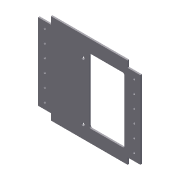
# Autodesk Inventor part: DriveTrain_MotorMount
Saved by Autodesk Inventor 2012 (Build 160160000, 160)
## iProperties
Created: 2012-01-08
Part Number: DriveTrain_MotorMount
Material: Aluminum-6061
Document SubType Name: Modeling
Designer: JesseK
Density: 2.71 g/cm^3
Mass: 300.27 g
Surface Area: 729.239 cm^2
Volume: 110.801 cm^3
Author: JesseK
Autodesk Inventor part; units mm, degrees
ref_plane "YZ Plane" through (0, 0, 0) normal (1, 0, 0) x (0, 1, 0)
ref_plane "XZ Plane" through (0, 0, 0) normal (0, 1, 0) x (-1, 0, 0)
ref_plane "XY Plane" through (0, 0, 0) normal (0, 0, 1) x (1, 0, 0)
sketch "Sketch1" plane through (0, 0, 0) normal (0, 0, 1) x (1, 0, 0)
  line L0 (203.2, 0) -> (203.2, 154.2919)
  line L1 (0, 152.4) -> (0, 0)
  line L2 (177.8, 154.2919) -> (177.8, 166.9919)
  line L3 (177.8, 166.9919) -> (25.4, 166.9919)
  line L4 (25.4, 166.9919) -> (25.4, 152.4)
  line L5 (0, 152.4) -> (25.4, 152.4)
  line L6 (177.8, 154.2919) -> (203.2, 154.2919)
  line L7 (177.8, 0) -> (177.8, -12.7)
  line L8 (177.8, -12.7) -> (25.4, -12.7)
  line L9 (25.4, -12.7) -> (25.4, 0)
  line L10 (0, 0) -> (25.4, 0)
  line L11 (177.8, 0) -> (203.2, 0)
  dimension "d0" = 152.4
  dimension "d1" = 203.2
  dimension "d18" = 25.4
  dimension "d19" = 25.4
  dimension "d20" = 12.7
  dimension "d21" = 25.4
  dimension "d22" = 25.4
  dimension "d23" = 12.7
  constraints: 24 end point, 4 parallel, 1 collinear, 1 perpendicular
  measures "d0" distance of L1.start L1.end
  measures "d1" distance of L1.end L0.start
  measures "d18" distance between parallel lines of L1 L4
  measures "d19" distance between parallel lines of L0 L2
  measures "d20" distance of L2.start L2.end
  measures "d21" distance of L1.end L9.end
  measures "d22" distance of L7.start L0.start
  measures "d23" distance of L7.start L7.end
extrude "Extrusion3" add sketch "Sketch1" along normal blind 3.175
sketch "Sketch2" plane through (0, 0, 3.175) normal (0, 0, 1) x (1, 0, 0)
  line L0 (0, 152.4) -> (25.4, 152.4) projected
  line L1 (0, 0) -> (0, 152.4) projected
  line L2 (25.4, 0) -> (0, 0) projected
  line L3 (203.2, 0) -> (177.8, 0) projected
  line L4 (177.8, 154.2919) -> (203.2, 154.2919) projected
  line L5 (25.4, 152.4) -> (25.4, 166.9919) projected
  line L6 (12.7, 152.4) -> (12.7, 139.7) construction
  line L7 (12.7, 139.7) -> (12.7, 114.3) construction
  line L8 (12.7, 114.3) -> (12.7, 88.9) construction
  line L9 (12.7, 88.9) -> (12.7, 63.5) construction
  line L10 (12.7, 63.5) -> (12.7, 38.1) construction
  line L11 (12.7, 38.1) -> (12.7, 12.7) construction
  line L12 (12.7, 12.7) -> (12.7, 0) construction
  circle A0 centre (12.7, 139.7) radius 2.3813
  circle A1 centre (12.7, 114.3) radius 2.3813
  circle A2 centre (12.7, 88.9) radius 2.3813
  circle A3 centre (12.7, 63.5) radius 2.3813
  circle A4 centre (12.7, 38.1) radius 2.3813
  circle A5 centre (12.7, 12.7) radius 2.3813
  line L13 (190.5, 154.2919) -> (190.5, 141.5919) construction
  line L14 (190.5, 141.5919) -> (190.5, 116.1919) construction
  line L15 (190.5, 116.1919) -> (190.5, 90.7919) construction
  line L16 (190.5, 90.7919) -> (190.5, 65.3919) construction
  line L17 (190.5, 65.3919) -> (190.5, 39.9919) construction
  line L18 (190.5, 39.9919) -> (190.5, 14.5919) construction
  line L19 (190.5, 14.5919) -> (190.5, 0) construction
  circle A6 centre (190.5, 141.5919) radius 2.3813
  circle A7 centre (190.5, 116.1919) radius 2.3813
  circle A8 centre (190.5, 90.7919) radius 2.3813
  circle A9 centre (190.5, 65.3919) radius 2.3813
  circle A10 centre (190.5, 39.9919) radius 2.3813
  circle A11 centre (190.5, 14.5919) radius 2.3813
  dimension "d26" = 12.7
  dimension "d27" = 25.4
  dimension "d28" = 4.7625
  dimension "d29" = 12.7
  dimension "d30" = 25.4
  dimension "d31" = 4.7625
  constraints: 28 end point, 18 collinear, 12 centre point, 12 coincident, 10 equal radius, 4 midpoint, 3 parallel
  measures "d26" distance of L6.start L6.end
  measures "d27" distance of L6.end L7.end
  measures "d28" diameter of A2
  measures "d29" distance of L13.start L13.end
  measures "d30" distance of L13.end L14.end
  measures "d31" diameter of A6
extrude "Extrusion4" cut sketch "Sketch2" against normal up to next
sketch "Sketch3" plane through (0, 0, 3.175) normal (0, 0, 1) x (1, 0, 0)
  line L0 (0, 0) -> (0, 152.4) projected
  line L1 (25.4, 0) -> (0, 0) projected
  circle A0 centre (88.9, 127) radius 3.175
  circle A1 centre (88.9, 12.7) radius 3.175
  dimension "d34" = 88.9
  dimension "d35" = 88.9
  dimension "d36" = 114.3
  dimension "d37" = 12.7
  dimension "d38" = 6.35
  dimension "d39" = 6.35
  constraints: 2 centre point
  measures "d34" distance from line of A0.centre L0
  measures "d35" distance from line of L0 A1.centre
  measures "d36" distance of A0.centre A1.centre
  measures "d37" distance from line of L1 A1.centre
  measures "d38" diameter of A0
  measures "d39" diameter of A1
extrude "Extrusion5" cut sketch "Sketch3" against normal up to next
sketch "Sketch4" plane through (0, 0, 3.175) normal (0, 0, 1) x (1, 0, 0)
  circle A0 centre (88.9, 127) radius 3.175 projected
  line L0 (203.2, 0) -> (177.8, 0) projected
  line L1 (203.2, 154.2919) -> (203.2, 0) projected
  line L2 (177.8, 154.2919) -> (203.2, 154.2919) projected
  line L3 (104.775, 141.5919) -> (168.275, 141.5919)
  line L4 (171.45, 138.4169) -> (171.45, 15.875)
  line L5 (168.275, 12.7) -> (104.775, 12.7)
  line L6 (101.6, 15.875) -> (101.6, 138.4169)
  arc A1 (104.775, 141.5919) -> (101.6, 138.4169) centre (104.775, 138.4169) ccw
  arc A2 (171.45, 138.4169) -> (168.275, 141.5919) centre (168.275, 138.4169) ccw
  arc A3 (168.275, 12.7) -> (171.45, 15.875) centre (168.275, 15.875) ccw
  arc A4 (101.6, 15.875) -> (104.775, 12.7) centre (104.775, 15.875) ccw
  dimension "d42" = 12.7
  dimension "d43" = 31.75
  dimension "d44" = 12.7
  dimension "d45" = 12.7
  dimension "d46" = 3.175
  constraints: 8 end point, 8 point on circle, 8 tangent, 4 centre point, 3 equal radius, 2 parallel, 1 horizontal, 1 perpendicular
  measures "d42" distance from line of L6 A0.centre
  measures "d43" distance between parallel lines of L1 L4
  measures "d44" distance between parallel lines of L2 L3
  measures "d45" distance between parallel lines of L0 L5
  measures "d46" radius of A1
extrude "Extrusion6" cut sketch "Sketch4" against normal up to next contours L3 A2 L4 A3 L5 A4 L6 A1
body "Solid3"
